Autodesk Fusion 360 part; units mm, degrees
(part 2 of 2)
sketch "Sketch2 (3)" plane through (-21, 0, 0) normal (1, 0, 0) x (0, 0, -1) in component "Wheels for tracks"
  line L0 (24.6356, 12.5534) -> (24.5049, 12.087)
  line L1 (24.5049, 12.087) -> (23.542, 12.3568)
  line L2 (23.542, 12.3568) -> (23.6727, 12.8232)
  arc A0 (23.6727, 12.8232) -> (22.5, 12.9844) centre (22, 5) ccw
  line L3 (22.5, 12.9844) -> (22.5, 12.5)
  line L4 (22.5, 12.5) -> (21.5, 12.5)
  line L5 (21.5, 12.5) -> (21.5, 12.9844)
  arc A1 (21.5, 12.9844) -> (20.3273, 12.8232) centre (22, 5) ccw
  line L6 (20.3273, 12.8232) -> (20.458, 12.3568)
  line L7 (20.458, 12.3568) -> (19.4951, 12.087)
  line L8 (19.4951, 12.087) -> (19.3644, 12.5534)
  arc A2 (19.3644, 12.5534) -> (18.2787, 12.0818) centre (22, 5) ccw
  line L9 (18.2787, 12.0818) -> (18.5303, 11.6679)
  line L10 (18.5303, 11.6679) -> (17.6759, 11.1484)
  line L11 (17.6759, 11.1484) -> (17.4242, 11.5622)
  arc A3 (17.4242, 11.5622) -> (16.506, 10.8152) centre (22, 5) ccw
  line L12 (16.506, 10.8152) -> (16.86, 10.4846)
  line L13 (16.86, 10.4846) -> (16.1775, 9.7537)
  line L14 (16.1775, 9.7537) -> (15.8235, 10.0843)
  arc A4 (15.8235, 10.0843) -> (15.1408, 9.1173) centre (22, 5) ccw
  line L15 (15.1408, 9.1173) -> (15.5709, 8.8944)
  line L16 (15.5709, 8.8944) -> (15.1108, 8.0065)
  line L17 (15.1108, 8.0065) -> (14.6808, 8.2294)
  arc A5 (14.6808, 8.2294) -> (14.2844, 7.114) centre (22, 5) ccw
  line L18 (14.2844, 7.114) -> (14.7586, 7.0155)
  line L19 (14.7586, 7.0155) -> (14.5551, 6.0364)
  line L20 (14.5551, 6.0364) -> (14.0809, 6.1349)
  arc A6 (14.0809, 6.1349) -> (14.0001, 4.954) centre (22, 5) ccw
  line L21 (14.0001, 4.954) -> (14.4834, 4.987)
  line L22 (14.4834, 4.987) -> (14.5516, 3.9893)
  line L23 (14.5516, 3.9893) -> (14.0684, 3.9563)
  arc A7 (14.0684, 3.9563) -> (14.3092, 2.7973) centre (22, 5) ccw
  line L24 (14.3092, 2.7973) -> (14.7656, 2.9595)
  line L25 (14.7656, 2.9595) -> (15.1005, 2.0173)
  line L26 (15.1005, 2.0173) -> (14.6441, 1.8551)
  arc A8 (14.6441, 1.8551) -> (15.1887, 0.8041) centre (22, 5) ccw
  line L27 (15.1887, 0.8041) -> (15.5844, 1.0834)
  line L28 (15.5844, 1.0834) -> (16.1611, 0.2664)
  line L29 (16.1611, 0.2664) -> (15.7654, -0.0129)
  arc A9 (15.7654, -0.0129) -> (16.5733, -0.878) centre (22, 5) ccw
  line L30 (16.5733, -0.878) -> (16.879, -0.5023)
  line L31 (16.879, -0.5023) -> (17.6547, -1.1334)
  line L32 (17.6547, -1.1334) -> (17.349, -1.5091)
  arc A10 (17.349, -1.5091) -> (18.3604, -2.1241) centre (22, 5) ccw
  line L33 (18.3604, -2.1241) -> (18.5534, -1.6799)
  line L34 (18.5534, -1.6799) -> (19.4706, -2.0783)
  line L35 (19.4706, -2.0783) -> (19.2776, -2.5225)
  arc A11 (19.2776, -2.5225) -> (20.4175, -2.8419) centre (22, 5) ccw
  line L36 (20.4175, -2.8419) -> (20.4834, -2.3621)
  line L37 (20.4834, -2.3621) -> (21.4741, -2.4982)
  line L38 (21.4741, -2.4982) -> (21.4081, -2.9781)
  arc A12 (21.4081, -2.9781) -> (22.5919, -2.9781) centre (22, 5) ccw
  line L39 (22.5919, -2.9781) -> (22.5259, -2.4982)
  line L40 (22.5259, -2.4982) -> (23.5166, -2.3621)
  line L41 (23.5166, -2.3621) -> (23.5825, -2.8419)
  arc A13 (23.5825, -2.8419) -> (24.7224, -2.5225) centre (22, 5) ccw
  line L42 (24.7224, -2.5225) -> (24.5294, -2.0783)
  line L43 (24.5294, -2.0783) -> (25.4466, -1.6799)
  line L44 (25.4466, -1.6799) -> (25.6396, -2.1241)
  arc A14 (25.6396, -2.1241) -> (26.651, -1.5091) centre (22, 5) ccw
  line L45 (26.651, -1.5091) -> (26.3453, -1.1334)
  line L46 (26.3453, -1.1334) -> (27.121, -0.5023)
  line L47 (27.121, -0.5023) -> (27.4267, -0.878)
  arc A15 (27.4267, -0.878) -> (28.2346, -0.0129) centre (22, 5) ccw
  line L48 (28.2346, -0.0129) -> (27.8389, 0.2664)
  line L49 (27.8389, 0.2664) -> (28.4156, 1.0834)
  line L50 (28.4156, 1.0834) -> (28.8113, 0.8041)
  arc A16 (28.8113, 0.8041) -> (29.3559, 1.8551) centre (22, 5) ccw
  line L51 (29.3559, 1.8551) -> (28.8995, 2.0173)
  line L52 (28.8995, 2.0173) -> (29.2344, 2.9595)
  line L53 (29.2344, 2.9595) -> (29.6908, 2.7973)
  arc A17 (29.6908, 2.7973) -> (29.9316, 3.9563) centre (22, 5) ccw
  line L54 (29.9316, 3.9563) -> (29.4484, 3.9893)
  line L55 (29.4484, 3.9893) -> (29.5166, 4.987)
  line L56 (29.5166, 4.987) -> (29.9999, 4.954)
  arc A18 (29.9999, 4.954) -> (29.9191, 6.1349) centre (22, 5) ccw
  line L57 (29.9191, 6.1349) -> (29.4449, 6.0364)
  line L58 (29.4449, 6.0364) -> (29.2414, 7.0155)
  line L59 (29.2414, 7.0155) -> (29.7156, 7.114)
  arc A19 (29.7156, 7.114) -> (29.3192, 8.2294) centre (22, 5) ccw
  line L60 (29.3192, 8.2294) -> (28.8892, 8.0065)
  line L61 (28.8892, 8.0065) -> (28.4291, 8.8944)
  line L62 (28.4291, 8.8944) -> (28.8592, 9.1173)
  arc A20 (28.8592, 9.1173) -> (28.1765, 10.0843) centre (22, 5) ccw
  line L63 (28.1765, 10.0843) -> (27.8225, 9.7537)
  line L64 (27.8225, 9.7537) -> (27.14, 10.4846)
  line L65 (27.14, 10.4846) -> (27.494, 10.8152)
  arc A21 (27.494, 10.8152) -> (26.5758, 11.5622) centre (22, 5) ccw
  line L66 (26.5758, 11.5622) -> (26.3241, 11.1484)
  line L67 (26.3241, 11.1484) -> (25.4697, 11.6679)
  line L68 (25.4697, 11.6679) -> (25.7213, 12.0818)
  arc A22 (25.7213, 12.0818) -> (24.6356, 12.5534) centre (22, 5) ccw
  circle A23 centre (22, 5) radius 2.1
  circle A24 centre (22, 5) radius 2.1
  circle A25 centre (22, 5) radius 1.5
  line L69 (23, 6.118) -> (23, 3.882)
  dimension "d136" = 1
  constraint concentric A24 A25
  constraint coincident A25 L69.start
  constraint coincident A25 L69.end
  constraint vertical L69
  measures "d136" distance of A0.centre L69
extrude "Extrude3'" add sketch "Sketch2 (3)" against normal blind 14 contours A23 A24 | A25 L69 picked at (23.1667, 5) bodies 7 in component "Wheels for tracks"
mirror "Mirror3''" about plane through (0, 0, 0) normal (1, 0, 0) of bodies 7 makes body 8 in component "Wheels for tracks"
sketch "Sketch1 (4)" plane through (0, 65, 0) normal (0, -1, 0) x (1, 0, 0)
  line L0 (43, -47) -> (47, -43)
  line L1 (47, -43) -> (47, 53.5)
  line L2 (47, 53.5) -> (-47, 53.5)
  line L3 (-47, 53.5) -> (-47, -43)
  line L4 (-47, -43) -> (-43, -47)
  line L5 (-43, -47) -> (43, -47)
  line L6 (28.75, -24.25) -> (-28.75, -24.25)
  line L7 (-28.75, -24.25) -> (-28.75, 24.25)
  line L8 (-28.75, 24.25) -> (28.75, 24.25)
  line L9 (28.75, 24.25) -> (28.75, -24.25)
  line L10 (28.75, -24.25) -> (-28.75, 24.25) construction
  line L11 (-28.75, -24.25) -> (28.75, 24.25) construction
  circle A0 centre (28.75, -24.25) radius 1.25
  circle A1 centre (28.75, -24.25) radius 3
  circle A2 centre (-28.75, -24.25) radius 1.25
  circle A3 centre (-28.75, -24.25) radius 3
  circle A4 centre (28.75, 24.25) radius 1.25
  circle A5 centre (28.75, 24.25) radius 3
  circle A6 centre (-28.75, 24.25) radius 1.25
  circle A7 centre (-28.75, 24.25) radius 3
  dimension "d141" = 57.5
  dimension "d142" = 48.5
  dimension "d143" = 2.5
  dimension "d144" = 6
  dimension "d145" = 2.5
  dimension "d146" = 6
  dimension "d147" = 2.5
  dimension "d148" = 6
  dimension "d149" = 2.5
  dimension "d150" = 6
  constraint horizontal L6
  constraint perpendicular L6 L7
  constraint parallel L6 L8
  constraint parallel L7 L9
  constraint coincident L10 origin
  constraint coincident L11 origin
  constraint coincident L6.start L9.end
  constraint concentric A0 A1
  constraint coincident L6.end L7.start
  constraint concentric A2 A3
  constraint coincident L8.end L9.start
  constraint concentric A4 A5
  constraint coincident L7.end L8.start
  constraint concentric A6 A7
  measures "d141" distance of L7.end L8.end
  measures "d142" distance of L6.end L7.end
  measures "d143" diameter of A0
  measures "d144" diameter of A1
  measures "d145" diameter of A2
  measures "d146" diameter of A3
  measures "d147" diameter of A4
  measures "d148" diameter of A5
  measures "d149" diameter of A6
  measures "d150" diameter of A7
extrude "Extrude9" add sketch "Sketch1 (4)" along normal blind 5 contours L6 L7 A2 A3 | L6 L7 A2 A3 | L6 L9 A0 A1 | L6 L9 A0 A1 | L7 L8 A6 A7 | L7 L8 A6 A7 | L8 L9 A4 A5 | L8 L9 A4 A5 bodies 2 in component "Top"
extrude "Extrude10" cut 4 faces at (-28.6185, 65, -25.1743) (28.4057, 65, -23.8911) (29.162, 65, 24.7547) (-28.4307, 65, 23.7817) along direction (0, 1, 0) blind 3 on bodies 2 bodies 2 in component "Top"
component "Bottom" placed x (1, 0, 0) y (0, 1, 0) z (0, 0, 1) at (0, 0, 0)
component "Top" placed x (1, 0, 0) y (0, 1, 0) z (0, 0, 1) at (0, 0, 0)
component "Wheels for tracks" placed x (1, 0, 0) y (0, 1, 0) z (0, 0, 1) at (0, 0, 0)
equation "d66 = d65"
